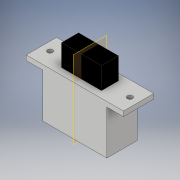
# Autodesk Inventor part: Switch
Saved by Autodesk Inventor 2019.4 (Build 234330000, 330)
## iProperties
Created: 2021-06-28
Part Number: Switch
Material: Generic
Document SubType Name: Modeling
Designer: keshav
Density: 1 g/cm^3
Appearance: Default
Author: keshav
Autodesk Inventor part; units mm, degrees
ref_plane "XZ Plane" through (0, 0, 0) normal (0, 1, 0) x (-1, 0, 0)
ref_plane "XY Plane" through (0, 0, 0) normal (0, 0, 1) x (1, 0, 0)
sketch "Sketch1" plane through (0, 0, 0) normal (0, 1, 0) x (-1, 0, 0)
  line L0 (-11.55, 3.6125) -> (11.55, 3.6125)
  line L1 (11.55, 3.6125) -> (11.55, -3.6125)
  line L2 (11.55, -3.6125) -> (-11.55, -3.6125)
  line L3 (-11.55, -3.6125) -> (-11.55, 3.6125)
  line L4 (-11.55, 3.6125) -> (11.55, -3.6125) construction
  line L5 (11.55, 3.6125) -> (-11.55, -3.6125) construction
  point P0 (0, 0)
  dimension "d0" = 23.1
  dimension "d1" = 7.225
  constraints: 12 end point, 2 midpoint, 2 parallel, 1 horizontal, 1 perpendicular
  measures "d0" distance of L1.end L2.end
  measures "d1" distance of L0.end L1.end
extrude "Extrusion1" add sketch "Sketch1" along normal blind 1.15
sketch "Sketch2" plane through (0, 0, 0) normal (0, -1, 0) x (1, 0, 0)
  line L0 (-11.55, 3.6125) -> (11.55, 3.6125) projected
  line L1 (-7.625, -3.6125) -> (7.625, -3.6125)
  line L2 (7.625, -3.6125) -> (7.625, 3.6125)
  line L3 (7.625, 3.6125) -> (-7.625, 3.6125)
  line L4 (-7.625, 3.6125) -> (-7.625, -3.6125)
  line L5 (-7.625, -3.6125) -> (7.625, 3.6125) construction
  line L6 (7.625, -3.6125) -> (-7.625, 3.6125) construction
  point P0 (0, 0)
  dimension "d4" = 15.25
  constraints: 12 end point, 2 midpoint, 2 parallel, 1 horizontal, 1 perpendicular, 1 point on line
  measures "d4" distance of L3.end L2.end
extrude "Extrusion2" add sketch "Sketch2" along normal blind 10.5
sketch "Sketch3" plane through (0, 1.15, 0) normal (0, 1, 0) x (1, 0, 0)
  line L0 (-4.75, -2.025) -> (4.75, -2.025)
  line L1 (4.75, -2.025) -> (4.75, 2.025)
  line L2 (4.75, 2.025) -> (-4.75, 2.025)
  line L3 (-4.75, 2.025) -> (-4.75, -2.025)
  line L4 (-4.75, -2.025) -> (4.75, 2.025) construction
  line L5 (4.75, -2.025) -> (-4.75, 2.025) construction
  point P0 (0, 0)
  dimension "d7" = 9.5
  dimension "d8" = 4.05
  constraints: 12 end point, 2 midpoint, 2 parallel, 1 horizontal, 1 perpendicular
  measures "d7" distance of L2.end L1.end
  measures "d8" distance between parallel lines of L0 L2
extrude "Extrusion3" add sketch "Sketch3" along normal blind 5.15
sketch "Sketch4" plane through (0, 1.15, 0) normal (0, 1, 0) x (1, 0, 0)
  line L0 (11.55, 3.6125) -> (-11.55, 3.6125) construction
  line L1 (0, 3.6125) -> (0, -3.6125) construction
  line L2 (-11.55, -3.6125) -> (11.55, -3.6125) construction
  line L3 (-11.55, 3.6125) -> (-11.55, -3.6125) construction
  line L4 (-11.55, 0) -> (11.55, 0) construction
  line L5 (11.55, -3.6125) -> (11.55, 3.6125) construction
  circle A0 centre (9.5, 0) radius 0.625
  circle A1 centre (-9.5, 0) radius 0.625
  point P0 (0, 0)
  dimension "d11" = 1.25
  dimension "d12" = 9.5
  constraints: 4 end point, 4 midpoint, 2 centre point, 1 point on line, 1 symmetric about line, 1 other
  measures "d11" diameter of A0
  measures "d12" distance from line of L1 A0.centre
extrude "Extrusion4" cut sketch "Sketch4" against normal up to surface (1.15 mm away)
body "Solid1"
